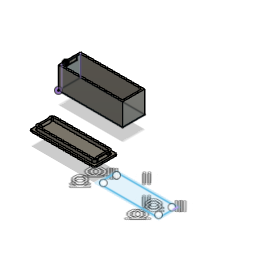
temperatureBox (Autodesk Fusion 360 design; units mm, degrees)
Autodesk Fusion 360 part; units mm, degrees
note: some values were not read from the file. Set by a fixed rule: which sketch regions a step uses.
sketch "Base" plane through (0, 0, 0) normal (0, 1, 0) x (1, 0, 0) in component "Top"
  line L0 (0, 0) -> (58, 0)
  line L1 (58, 0) -> (58, 20)
  line L2 (58, 20) -> (0, 20)
  line L3 (0, 20) -> (0, 0)
  dimension "d6" = 58
  dimension "d7" = 20
  constraint horizontal L0
  constraint vertical L1
  constraint horizontal L2
  constraint vertical L3
  constraint coincident L0.start L3.end
  measures "d6" distance of L0.start L0.end
  measures "d7" distance of L0.start L2.end
extrude "Extrude1" add sketch "Base" along normal blind 20 makes body 1 in component "Top"
shell "Shell1" thickness 1.5 removed faces 1 at (19.3333, 20, -13.3333) on bodies 1 in component "Top"
sketch "Knob" plane through (1.5, 0, 0) normal (1, 0, 0) x (0, 0, -1) in component "Top"
  line L0 (18.5, 20) -> (1.5, 20)
  line L1 (1.5, 1.5) -> (18.5, 1.5)
  line L2 (5, 20) -> (15, 20)
  line L3 (15, 20) -> (15, 17)
  line L4 (15, 17) -> (5, 17)
  line L5 (5, 17) -> (5, 20)
  line L6 (10, 20) -> (10, 17) construction
  line L7 (18.5, 1.5) -> (18.5, 20)
  line L8 (1.5, 20) -> (1.5, 1.5)
  dimension "d12" = 10
  dimension "d13" = 3
  constraint horizontal L2
  constraint vertical L3
  constraint horizontal L4
  constraint vertical L5
  constraint coincident L0 L2.start
  constraint midpoint L0 L6.start
  constraint midpoint L4 L6.end
  constraint vertical L6
  measures "d12" distance of L3.end L4.end
  measures "d13" distance of L2.end L3.end
extrude "Extrude2" add sketch "Knob" along normal blind 6 draft -45 contours L0 L2 L3 L4 L5 bodies 1 in component "Top"
ref_plane "WorkPlane2" through (29, 10, -10) normal (-1, 0, 0) x (0, 0, 1) in component "Top"
mirror "Mirror1" about plane through (29, 10, -10) normal (-1, 0, 0) of "Extrude2" in component "Top"
sketch "Top" plane through (0, 20, 0) normal (0, 1, 0) x (-1, 0, 0) in component "Base"
  line L0 (-58, 0) -> (-58, -20)
  line L1 (-58, -20) -> (0, -20)
  line L2 (0, -20) -> (0, 0)
  line L3 (0, 0) -> (-58, 0)
  line L4 (-56.5, -5) -> (-56.5, -1.5)
  line L5 (-56.5, -1.5) -> (-1.5, -1.5)
  line L6 (-1.5, -1.5) -> (-1.5, -5)
  line L7 (-1.5, -5) -> (-1.5, -15)
  line L8 (-1.5, -15) -> (-1.5, -18.5)
  line L9 (-1.5, -18.5) -> (-56.5, -18.5)
  line L10 (-56.5, -15) -> (-56.5, -5)
  line L11 (-56.5, -18.5) -> (-56.5, -15)
extrude "Extrude1'" add sketch "Top" along normal blind 1.5 separate body contours L0 L1 L2 L3 | L4 L5 L6 L7 L8 L9 L10 L11 makes body 2 in component "Base"
sketch "Lip" plane through (0, 20, 0) normal (0, -1, 0) x (1, 0, 0) in component "Base"
  line L0 (58, 0) -> (0, 0)
  line L1 (0, 0) -> (0, -20)
  line L2 (0, -20) -> (58, -20)
  line L3 (58, -20) -> (58, 0)
  line L4 (56.3, -16) -> (56.3, -4)
  arc A0 (56.3, -4) -> (54, -1.7) centre (54, -4) ccw
  line L5 (54, -1.7) -> (4, -1.7)
  arc A1 (4, -1.7) -> (1.7, -4) centre (4, -4) ccw
  line L6 (1.7, -4) -> (1.7, -16)
  arc A2 (1.7, -16) -> (4, -18.3) centre (4, -16) ccw
  line L7 (4, -18.3) -> (54, -18.3)
  arc A3 (54, -18.3) -> (56.3, -16) centre (54, -16) ccw
  constraint parallel L3 L4
  constraint parallel L0 L5
  constraint parallel L1 L6
  constraint parallel L2 L7
  constraint tangent L4 A0
  constraint tangent L4 A3
  constraint tangent A2 L7
  constraint tangent L5 A1
  constraint tangent A0 L5
  constraint tangent A1 L6
  constraint tangent L6 A2
  constraint tangent L7 A3
extrude "Extrude2'" add sketch "Lip" along normal blind 3 contours L4 A0 L5 A1 L6 A2 L7 A3 bodies 2 in component "Base"
extrude "Extrude3" cut sketch "Knob" along normal blind 3 draft -45 from surface at 0.2 contours L0 L2 L3 L4 L5 bodies 2 in component "Base"
mirror "Mirror1'" about plane through (29, 10, -10) normal (-1, 0, 0) of "Extrude3" in component "Base"
shell "Shell1'" thickness 1.5 removed faces 1 at (37.3333, 17, -12.7667) on bodies 2 in component "Base"
chamfer "Chamfer1" distance 0.6 angle 45 2 edges at (1.7, 17, -10) (56.3, 17, -10) on bodies 2 in component "Base"
move_body "Move1" bodies 2 to x (-1, 0, 0) y (0, -1, 0) z (0, 0, 1) at (0, 53, 0) in component "Base"
component "Enclosure" placed x (1, 0, 0) y (0, 1, 0) z (0, 0, 1) at (0, 0, 0)
component "Top" placed x (1, 0, 0) y (0, 1, 0) z (0, 0, 1) at (0, 0, 0) in component "Enclosure"
component "Base" placed x (1, 0, 0) y (0, 1, 0) z (0, 0, 1) at (0, 0, 0) in component "Enclosure"
equation "Width = 20 mm"
equation "length = 58 mm"
equation "heigth = 20 mm"
equation "shell = 1.5 mm"
equation "gap = 0.2 mm"
equation "d6 = length"
equation "d7 = Width"
equation "d8 = heigth"
equation "d11 = shell"
equation "d12 = Width / 2"
equation "d13 = shell * 2"
equation "d17 = shell"
equation "d20 = shell * 2"
equation "d23 = shell * 2"
equation "d26 = shell"
